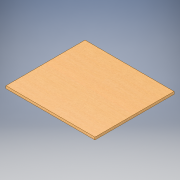
# Autodesk Inventor part: Tun-Platform
Saved by Autodesk Inventor 2017 (Build 210142000, 142)
## iProperties
Created: 2017-08-30
Part Number: Tun-Platform
Material: Generic
Document SubType Name: Modeling
Designer: Trent
Density: 1 g/cm^3
Appearance: Yellow Pine - Solid Stained Light Low Gloss
Author: Trent
Autodesk Inventor part; units mm, degrees
ref_plane "YZ Plane" through (0, 0, 0) normal (1, 0, 0) x (0, 1, 0)
ref_plane "XZ Plane" through (0, 0, 0) normal (0, 1, 0) x (-1, 0, 0)
ref_plane "XY Plane" through (0, 0, 0) normal (0, 0, 1) x (1, 0, 0)
sketch "Sketch1" plane through (0, 0, 0) normal (0, 1, 0) x (-1, 0, 0)
  line L0 (228.6, 203.2) -> (-228.6, 203.2)
  line L1 (-228.6, 203.2) -> (-228.6, -203.2)
  line L2 (-228.6, -203.2) -> (228.6, -203.2)
  line L3 (228.6, -203.2) -> (228.6, 203.2)
  line L4 (228.6, 203.2) -> (-228.6, -203.2) construction
  line L5 (-228.6, 203.2) -> (228.6, -203.2) construction
  point P0 (0, 0)
  dimension "d0" = 457.2
  dimension "d1" = 406.4
  constraints: 12 end point, 2 midpoint, 2 parallel, 1 horizontal, 1 perpendicular
  measures "d0" distance of L2.end L1.end
  measures "d1" distance of L1.end L0.end
extrude "Extrusion1" add sketch "Sketch1" along normal blind 12.7
body "Solid1"
